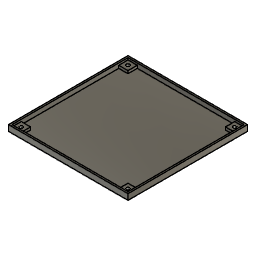
Junu_Arduino_Base_V1 (Autodesk Fusion 360 design; units mm, degrees)
part number: 2025-07-12-15-34-12-089
Autodesk Fusion 360 part; units mm, degrees
sketch "스케치1" plane through (0, 0, 0) normal (0, 0, 1) x (1, 0, 0)
  line L0 (0, 0) -> (103, 0)
  line L1 (103, 0) -> (103, 103)
  line L2 (103, 103) -> (0, 103)
  line L3 (0, 103) -> (0, 0)
  line L4 (0, 80.7838) -> (1.5, 80.7838)
  line L5 (4.5156, 103) -> (4.5156, 101.5)
  line L6 (1.5, 101.5) -> (101.5, 101.5)
  line L7 (101.5, 101.5) -> (101.5, 1.5)
  line L8 (101.5, 1.5) -> (1.5, 1.5)
  line L9 (1.5, 1.5) -> (1.5, 101.5)
  line L10 (1.5, 101.5) -> (9.5, 101.5)
  line L11 (9.5, 101.5) -> (9.5, 93.5)
  line L12 (9.5, 93.5) -> (1.5, 93.5)
  line L13 (1.5, 93.5) -> (1.5, 101.5)
  line L14 (1.5, 1.5) -> (9.5, 1.5)
  line L15 (9.5, 1.5) -> (9.5, 9.5)
  line L16 (9.5, 9.5) -> (1.5, 9.5)
  line L17 (1.5, 9.5) -> (1.5, 1.5)
  line L18 (101.5, 1.5) -> (93.5, 1.5)
  line L19 (93.5, 1.5) -> (93.5, 9.5)
  line L20 (93.5, 9.5) -> (101.5, 9.5)
  line L21 (101.5, 9.5) -> (101.5, 1.5)
  line L22 (101.5, 101.5) -> (93.5, 101.5)
  line L23 (93.5, 101.5) -> (93.5, 93.5)
  line L24 (93.5, 93.5) -> (101.5, 93.5)
  line L25 (101.5, 93.5) -> (101.5, 101.5)
  circle A0 centre (5.5, 97.5) radius 1.5
  circle A1 centre (97.5, 97.5) radius 1.4
  circle A2 centre (5.5, 5.5) radius 1.4
  circle A3 centre (97.5, 5.5) radius 1.5
  dimension "d1" = 103
  dimension "d5" = 100
  dimension "d6" = 100
  dimension "d7" = 1.5
  dimension "d8" = 1.5
  dimension "d9" = 1.5
  dimension "d10" = 8
  dimension "d11" = 8
  dimension "d12" = 8
  dimension "d13" = 8
  dimension "d14" = 8
  dimension "d15" = 8
  dimension "d16" = 8
  dimension "d17" = 8
  dimension "d18" = 3
  dimension "d20" = 4
  dimension "d21" = 4
  dimension "d22" = 2.8
  dimension "d23" = 4
  dimension "d24" = 4
  dimension "d25" = 2.8
  dimension "d26" = 4
  dimension "d27" = 4
  dimension "d28" = 3
  dimension "d29" = 4
  dimension "d30" = 4
  constraint horizontal L0
  constraint vertical L1
  constraint horizontal L2
  constraint vertical L3
  constraint coincident L0.start L3.end
  constraint coincident L3 L4.start
  constraint horizontal L4
  constraint coincident L2 L5.start
  constraint perpendicular L2 L5
  constraint horizontal L6
  constraint vertical L7
  constraint horizontal L8
  constraint vertical L9
  constraint horizontal L10
  constraint vertical L11
  constraint horizontal L12
  constraint vertical L13
  constraint horizontal L14
  constraint vertical L15
  constraint horizontal L16
  constraint vertical L17
  constraint horizontal L18
  constraint vertical L19
  constraint horizontal L20
  constraint vertical L21
  constraint horizontal L22
  constraint vertical L23
  constraint horizontal L24
  constraint vertical L25
  measures "d1" distance of L0.start L0.end
  measures "d5" distance of L6.start L6.end
  measures "d6" distance of L6.start L8.end
  measures "d7" distance of L2 L6
  measures "d8" distance of L3 L9
  measures "d9" distance of L0 L8
  measures "d10" distance of L6.start L10.end
  measures "d11" distance of L6.start L12.end
  measures "d12" distance of L8.end L14.end
  measures "d13" distance of L8.end L16.end
  measures "d14" distance of L7.end L18.end
  measures "d15" distance of L7.end L20.end
  measures "d16" distance of L6.end L22.end
  measures "d17" distance of L6.end L24.end
  measures "d18" diameter of A0
  measures "d20" distance of L10 A0.centre
  measures "d21" distance of L13 A0.centre
  measures "d22" diameter of A1
  measures "d23" distance of L7 A1.centre
  measures "d24" distance of L6 A1.centre
  measures "d25" diameter of A2
  measures "d26" distance of L8 A2.centre
  measures "d27" distance of L17 A2.centre
  measures "d28" diameter of A3
  measures "d29" distance of L21 A3.centre
  measures "d30" distance of L18 A3.centre
extrude "돌출1" add sketch "스케치1" along normal blind 5 contours L0 L1 L2 L3 L4 L5 L6 L7 L8 L9 L10 L14 L17 L18 L21 L22 L25 | L2 L3 L4 L5 L6 L9 L10 L13
extrude "돌출2" add sketch "스케치1" along normal blind 3.3 contours L8 L9 L14 L15 L16 L17 | L6 L9 L10 L11 L12 L13 | L6 L7 L22 L23 L24 L25 | L7 L8 L18 L19 L20 L21
extrude "돌출3" add sketch "스케치1" along normal blind 1 contours L6 L7 L8 L9 L11 L12 L15 L16 L19 L20 L23 L24
extrude "돌출4" add sketch "스케치1" along normal blind 1 contours A0 | A1 | A2 | A3
